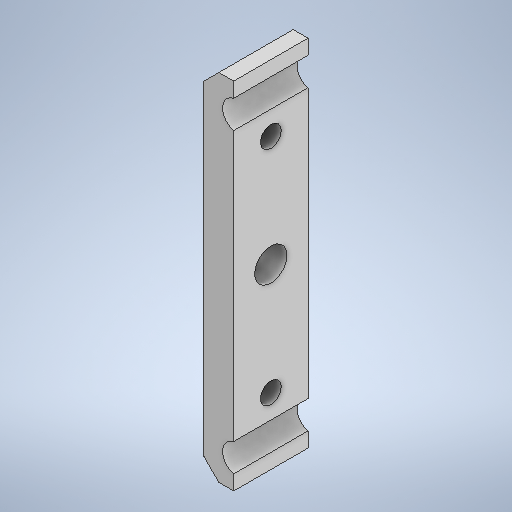
# Autodesk Inventor part: 6xMounting_clamp
Saved by Autodesk Inventor 2025.1 (Build 291241020, 241B)
## iProperties
Created: 2024-11-24
Part Number: 6xMounting_clamp
Material: Ogólny
Document SubType Name: Modeling
Designer: zychlix
Density: 1 g/cm^3
Appearance: Domyślna
Author: zychlix
Autodesk Inventor part; units mm, degrees
ref_plane "YZ Plane" through (0, 0, 0) normal (1, 0, 0) x (0, 1, 0)
ref_plane "XZ Plane" through (0, 0, 0) normal (0, 1, 0) x (-1, 0, 0)
ref_plane "XY Plane" through (0, 0, 0) normal (0, 0, 1) x (1, 0, 0)
sketch "Szkic1" plane through (0, 0, 0) normal (0, 0, 1) x (1, 0, 0)
  circle A0 centre (0, 30) radius 3 construction
  arc A1 (-0.6454, 32.8273) -> (-0.6454, 27.1727) centre (0, 30) ccw
  line L0 (-0.6454, 27.1727) -> (-0.6454, 0)
  line L1 (-0.6454, 32.8273) -> (-0.6454, 35.8273)
  line L2 (-0.6454, 35.8273) -> (-3.6454, 35.8273)
  line L3 (-3.6454, 35.8273) -> (-6.6454, 32.8273)
  line L4 (-6.6454, 32.8273) -> (-6.6454, 0)
  line L5 (-0.6454, 0) -> (-6.6454, 0)
  point P0 (0, 0)
  dimension "d0" = 6
  dimension "d1" = 30
  dimension "d2" = 5.8
  dimension "d3" = 3
  dimension "d4" = 45
  dimension "d5" = 3
  dimension "d6" = 3
  constraints: 12 end point, 2 centre point, 2 point on circle, 1 coincident, 1 collinear, 1 horizontal, 1 parallel, 1 perpendicular, 1 point on line, 1 vertical
  measures "d0" diameter of A0
  measures "d1" distance of point (0, 0) A0.centre
  measures "d2" diameter of A1
  measures "d3" distance from line of L1.start L2
  measures "d4" angle of L2 L3
  measures "d5" distance from line of L4 L2.end
  measures "d6" distance of L1.end L2.end
extrude "Wyciągnięcie proste1" add sketch "Szkic1" along normal blind 15
sketch "Szkic2" plane through (-6.6454, 0, 0) normal (-1, 0, 0) x (0, 0, 1)
  circle A0 centre (7.5, 22.3961) radius 2.1
  line L0 (0, 32.8273) -> (15, 32.8273) projected
  point P0 (0, 0)
  point P1 (7.5, 32.8273)
  dimension "d9" = 4.2
  constraints: 1 centre point, 1 midpoint, 1 vertical alignment
  measures "d9" diameter of A0
extrude "Wyciągnięcie proste2" cut sketch "Szkic2" against normal blind 8
mirror "Odbij1" about plane through (-6.6454, 0, 0) normal (0, -1, 0) of "Wyciągnięcie proste1", "Wyciągnięcie proste2"
sketch "Szkic3" plane through (-6.6454, 32.8273, 0) normal (-1, 0, 0) x (0, 0, 1)
  circle A0 centre (7.5, -32.8273) radius 3.25
  line L0 (0, 3) -> (15, 3) projected
  line L1 (0, 0) -> (0, -65.6545) projected
  point P0 (0, -32.8273)
  point P1 (7.5, 3)
  point P2 (0, -32.8273)
  point P3 (0, -32.8273)
  dimension "d12" = 6.5
  constraints: 3 midpoint, 2 horizontal alignment, 1 centre point, 1 vertical alignment
  measures "d12" diameter of A0
extrude "Wyciągnięcie proste3" cut sketch "Szkic3" against normal through all
